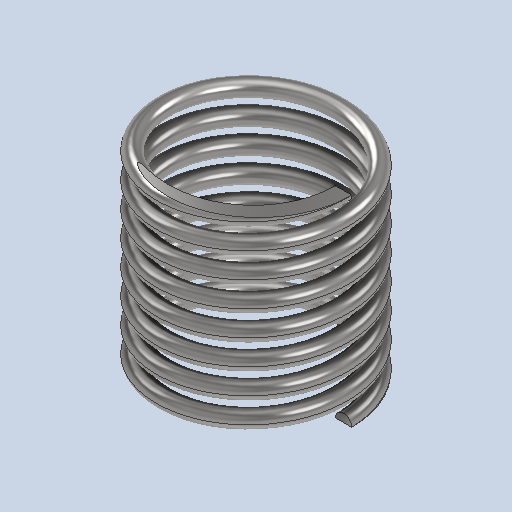
# Autodesk Inventor part: Spring
Saved by Autodesk Inventor 2022 (Build 260153000, 153)
## iProperties
Created: 2020-03-11
Part Number: Spring
Material: Stainless Steel
Document SubType Name: Modeling
Designer: elmar
Density: 8 g/cm^3
Appearance: Semi-Polished
Author: elmar
Autodesk Inventor part; units mm, degrees
ref_plane "YZ Plane" through (0, 0, 0) normal (1, 0, 0) x (0, 1, 0)
ref_plane "XZ Plane" through (0, 0, 0) normal (0, 1, 0) x (-1, 0, 0)
sketch "Sketch1" plane through (0, 0, 0) normal (0, 0, 1) x (1, 0, 0)
  line L0 (-0.9525, 0) -> (5.715, 0) projected
  circle A0 centre (4.3561, 0) radius 0.4064
  point P0 (0, 0)
  point P1 (4.7625, 0)
  dimension "d0" = 0.8128
  dimension "d10" = 4.7625
  constraints: 1 horizontal alignment, 1 point on line, 2 other
  measures "d10" distance of point (0, 0) point (4.763, 0)
coil "Coil1" sketch "Sketch1" operation add axis through (0, -10, 0) along (0, -1, 0) pitch 1.25 turns 8 hand right
ref_plane "Work Plane1" through (4.7625, -10, 0) normal (0, 1, 0) x (-1, 0, 0)
split "Split1" plane through (4.7625, -10, 0) removes the side toward (0, -1, 0)
split "Split2" plane through (0, 0, 0) removes the side toward (0, 1, 0)
body "Solid1"
